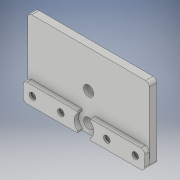
# Autodesk Inventor part: HX711MountingBracket
Saved by Autodesk Inventor 2019.3 (Build 233278000, 278)
## iProperties
Created: 2019-02-11
Part Number: HX711MountingBracket
Material: Generic
Document SubType Name: Modeling
Designer: mark
Density: 1 g/cm^3
Appearance: Default
Author: mark
Autodesk Inventor part; units mm, degrees
ref_plane "YZ Plane" through (0, 0, 0) normal (1, 0, 0) x (0, 1, 0)
ref_plane "XZ Plane" through (0, 0, 0) normal (0, 1, 0) x (-1, 0, 0)
ref_plane "XY Plane" through (0, 0, 0) normal (0, 0, 1) x (1, 0, 0)
sketch "Sketch1" plane through (0, 0, 0) normal (0, 0, 1) x (1, 0, 0)
  line L0 (0, 0) -> (65, 0)
  line L1 (65, 0) -> (65, 40)
  line L2 (65, 40) -> (0, 40)
  line L3 (0, 40) -> (0, 0)
  circle A0 centre (32.5, 5) radius 2.75
  circle A1 centre (32.5, 20) radius 2.75
  arc A2 (2.354249, 8) -> (2.354249, 2) centre (5, 5) ccw
  arc A3 (17.554249, 8) -> (17.554249, 2) centre (20.2, 5) ccw
  line L4 (2.354249, 8) -> (7.645751, 8)
  line L5 (2.354249, 2) -> (7.645751, 2)
  arc A4 (7.645751, 2) -> (7.645751, 8) centre (5, 5) ccw
  line L6 (17.554249, 8) -> (22.845751, 8)
  line L7 (17.554249, 2) -> (22.845751, 2)
  arc A5 (22.845751, 2) -> (22.845751, 8) centre (20.2, 5) ccw
  arc A6 (42.154249, 8) -> (42.154249, 2) centre (44.8, 5) ccw
  arc A7 (57.354249, 8) -> (57.354249, 2) centre (60, 5) ccw
  line L8 (42.154249, 8) -> (47.445751, 8)
  line L9 (42.154249, 2) -> (47.445751, 2)
  line L10 (57.354249, 2) -> (62.645751, 2)
  line L11 (57.354249, 8) -> (62.645751, 8)
  arc A8 (47.445751, 2) -> (47.445751, 8) centre (44.8, 5) ccw
  arc A9 (62.645751, 2) -> (62.645751, 8) centre (60, 5) ccw
  dimension "d0" = 65
  dimension "d1" = 40
  dimension "d14" = 5.5
  dimension "d15" = 5.5
  dimension "d16" = 5
  dimension "d17" = 20
  dimension "d18" = 32.5
  dimension "d19" = 32.5
  dimension "d59" = 15.2
  dimension "d60" = 5
  dimension "d61" = 5
  dimension "d62" = 5
  dimension "d65" = 3
  dimension "d66" = 6
  dimension "d67" = 3
  dimension "d68" = 6
  dimension "d69" = 4
  dimension "d70" = 4
  dimension "d73" = 5
  dimension "d74" = 5
  dimension "d75" = 5
  dimension "d76" = 15.2
  dimension "d77" = 3
  dimension "d78" = 6
  dimension "d79" = 3
  dimension "d80" = 6
  dimension "d81" = 4
  dimension "d82" = 4
  constraints: 24 end point, 20 point on circle, 10 centre point, 10 horizontal, 2 vertical
  measures "d0" distance between parallel lines of L1 L3
  measures "d1" distance between parallel lines of L0 L2
  measures "d14" diameter of A0
  measures "d15" diameter of A1
  measures "d16" distance from line of L0 A0.centre
  measures "d17" distance from line of L2 A1.centre
  measures "d18" distance from line of L3 A1.centre
  measures "d19" distance from line of L3 A0.centre
  measures "d59" distance of A3.centre A2.centre
  measures "d60" distance from line of L0 A3.centre
  measures "d61" distance from line of L0 A2.centre
  measures "d62" distance from line of L3 A2.centre
  measures "d65" distance from line of A2.centre L4
  measures "d66" distance between parallel lines of L5 L4
  measures "d67" distance from line of L6 A3.centre
  measures "d68" distance between parallel lines of L7 L6
  measures "d69" radius of A5
  measures "d70" radius of A4
  measures "d73" distance from line of L1 A7.centre
  measures "d74" distance from line of L0 A7.centre
  measures "d75" distance from line of L0 A6.centre
  measures "d76" distance of A7.centre A6.centre
  measures "d77" distance from line of A6.centre L8
  measures "d78" distance between parallel lines of L9 L8
  measures "d79" distance from line of A7.centre L11
  measures "d80" distance between parallel lines of L11 L10
  measures "d81" radius of A8
  measures "d82" radius of A9
sketch "Sketch1 outline for Extrusion2" plane through (0, 0, 0) normal (0, 0, 1) x (1, 0, 0)
  line L0 (0, 40) -> (0, 0)
  line L1 (65, 40) -> (0, 40)
  line L2 (0, 0) -> (65, 0)
  line L3 (65, 0) -> (65, 40)
  line L4 (7.645751, 8) -> (2.354249, 8)
  arc A0 (2.354249, 8) -> (2.354249, 2) centre (5, 5) ccw
  line L5 (2.354249, 2) -> (7.645751, 2)
  arc A1 (7.645751, 2) -> (7.645751, 8) centre (5, 5) ccw
  line L6 (22.845751, 8) -> (17.554249, 8)
  arc A2 (17.554249, 8) -> (17.554249, 2) centre (20.2, 5) ccw
  line L7 (17.554249, 2) -> (22.845751, 2)
  arc A3 (22.845751, 2) -> (22.845751, 8) centre (20.2, 5) ccw
  circle A4 centre (32.5, 5) radius 2.75
  line L8 (47.445751, 8) -> (42.154249, 8)
  arc A5 (42.154249, 8) -> (42.154249, 2) centre (44.8, 5) ccw
  line L9 (42.154249, 2) -> (47.445751, 2)
  arc A6 (47.445751, 2) -> (47.445751, 8) centre (44.8, 5) ccw
  arc A7 (57.354249, 8) -> (57.354249, 2) centre (60, 5) ccw
  line L10 (57.354249, 2) -> (62.645751, 2)
  arc A8 (62.645751, 2) -> (62.645751, 8) centre (60, 5) ccw
  line L11 (62.645751, 8) -> (57.354249, 8)
  circle A9 centre (32.5, 20) radius 2.75
extrude "Extrusion2" add sketch "Sketch1 outline for Extrusion2" along normal blind 4
sketch "Sketch3" plane through (0, 0, 4) normal (0, 0, 1) x (1, 0, 0)
  arc A0 (6.430909, 2.25) -> (6.430909, 7.75) centre (5, 5) ccw
  arc A1 (21.630909, 2.25) -> (21.630909, 7.75) centre (20.2, 5) ccw
  arc A2 (46.230909, 2.25) -> (46.230909, 7.75) centre (44.8, 5) ccw
  arc A3 (61.430909, 2.25) -> (61.430909, 7.75) centre (60, 5) ccw
  circle A4 centre (5, 5) radius 1.75
  circle A5 centre (20.2, 5) radius 1.75
  circle A6 centre (44.8, 5) radius 1.75
  circle A7 centre (60, 5) radius 1.75
  line L0 (-0.001228, 10) -> (65.024294, 10)
  line L1 (0, 0) -> (65, 0)
  line L2 (0, 40) -> (0, 0)
  line L3 (-0.001228, 10) -> (0, 0)
  line L4 (0, 0) -> (65, 0)
  line L5 (65, 0) -> (65, 40)
  line L6 (65.024294, 10) -> (65, 0)
  circle A8 centre (32.5, 5) radius 2.75
  circle A9 centre (32.5, 5) radius 5.25
  dimension "d37" = 3.5
  dimension "d38" = 3.5
  dimension "d39" = 3.5
  dimension "d40" = 3.5
  dimension "d45" = 10
  dimension "d49" = 10.5
  constraints: 8 end point, 5 centre point, 5 coincident, 1 horizontal
  measures "d37" diameter of A7
  measures "d38" diameter of A6
  measures "d39" diameter of A5
  measures "d40" diameter of A4
  measures "d45" distance between parallel lines of L1 L0
  measures "d49" diameter of A9
sketch "Sketch3 outline for Extrusion3" plane through (0, 0, 4) normal (0, 0, 1) x (1, 0, 0)
  line L0 (30.899219, 10) -> (-0.001228, 10)
  arc A0 (30.899219, 10) -> (30.899219, 0) centre (32.5, 5) ccw
  line L1 (0, 0) -> (30.899219, 0)
  line L2 (-0.001228, 10) -> (0, 0)
  circle A1 centre (5, 5) radius 1.75
  circle A2 centre (20.2, 5) radius 1.75
  line L3 (65.024294, 10) -> (34.100781, 10)
  arc A3 (34.100781, 10) -> (34.100781, 0) centre (32.5, 5) cw
  line L4 (34.100781, 0) -> (65, 0)
  line L5 (65, 0) -> (65.024294, 10)
  circle A4 centre (44.8, 5) radius 1.75
  circle A5 centre (60, 5) radius 1.75
extrude "Extrusion3" add sketch "Sketch3 outline for Extrusion3" along normal blind 2.5
fillet "Fillet1" radius 2 6 edges at (0, 0, 5.25) (65, 0, 5.25) (65, 40, 2) (0, 40, 2) (-0.0012, 10, 5.25) (65.0243, 10, 5.25)
chamfer "Chamfer1" distance 1.5 angle 45 4 edges at (58.25, 5, 4) (43.05, 5, 4) (18.45, 5, 4) (3.25, 5, 4)
chamfer "Chamfer2" distance 2 angle 45 4 edges at (34.1008, 0, 5.25) (30.8992, 0, 5.25) (30.8992, 10, 5.25) (34.1008, 10, 5.25)
body "Solid2"
